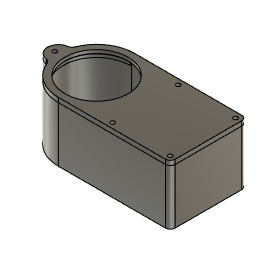
ad_extbox_alarm v14 (Autodesk Fusion 360 design; units mm, degrees)
Autodesk Fusion 360 part; units mm, degrees
note: some values were not read from the file. Set by a fixed rule: which face or edge a step refers to.
sketch "Sketch1" plane through (0, 0, 0) normal (0, 0, 1) x (1, 0, 0)
  circle A0 centre (0, 0) radius 31.5
  line L0 (-0.0628, 31.4999) -> (92.4372, 31.4999)
  line L1 (92.4372, 31.4999) -> (92.4372, -31.5001)
  line L2 (92.4372, -31.5001) -> (-0.0628, -31.5001)
  line L3 (-0.0628, -31.5001) -> (-0.0628, 31.4999)
  circle A1 centre (71.4372, -0.0001) radius 11
  circle A2 centre (26.4372, 24.9999) radius 1.75
  circle A3 centre (26.4372, -25.0001) radius 1.75
  circle A4 centre (71.4372, -25.0001) radius 1.75
  circle A5 centre (71.4372, 24.9999) radius 1.75
  circle A6 centre (0, 0) radius 26.15
  circle A7 centre (92.4372, 31.4999) radius 10.8
  circle A8 centre (92.4372, -31.5001) radius 10.8
  circle A9 centre (40.4372, -31.5001) radius 9
  circle A10 centre (40.4372, 31.4999) radius 9
  line L4 (40.4372, 26.9999) -> (87.9372, 26.9999)
  line L5 (87.9372, 26.9999) -> (87.9372, -27.0001)
  line L6 (87.9372, -27.0001) -> (40.4372, -27.0001)
  line L7 (40.4372, -27.0001) -> (40.4372, 26.9999)
  circle A11 centre (40.4372, -27.0001) radius 1.75
  circle A12 centre (87.9372, -27.0001) radius 1.75
  circle A13 centre (87.9372, 26.9999) radius 1.75
  circle A14 centre (40.4372, 26.9999) radius 1.75
  line L8 (57.4372, -24.8001) -> (77.4372, -24.8001)
  line L9 (77.4372, -24.8001) -> (77.4372, -28.8001)
  line L10 (77.4372, -28.8001) -> (57.4372, -28.8001)
  line L11 (57.4372, -28.8001) -> (57.4372, -24.8001)
  line L12 (57.4372, 28.7999) -> (77.4372, 28.7999)
  line L13 (77.4372, 28.7999) -> (77.4372, 24.7999)
  line L14 (77.4372, 24.7999) -> (57.4372, 24.7999)
  line L15 (57.4372, 24.7999) -> (57.4372, 28.7999)
  line L16 (85.7372, 9.9999) -> (89.7372, 9.9999)
  line L17 (89.7372, 9.9999) -> (89.7372, -10.0001)
  line L18 (89.7372, -10.0001) -> (85.7372, -10.0001)
  line L19 (85.7372, -10.0001) -> (85.7372, 9.9999)
  circle A15 centre (0, 0) radius 28.8
  circle A16 centre (0, 0) radius 27.75
  circle A17 centre (-31.5, 0.013) radius 9
  circle A18 centre (-34.5, 0.0043) radius 1.75
  circle A19 centre (-34.5, 0.0043) radius 2
  circle A20 centre (40.4372, 26.9999) radius 2
  circle A21 centre (87.9372, 26.9999) radius 2
  circle A22 centre (87.9372, -27.0001) radius 2
  circle A23 centre (40.4372, -27.0001) radius 2
  dimension "d1" = 63
  dimension "d6" = 92.5
  dimension "d7" = 63
  dimension "d8" = 22
  dimension "d9" = 21
  dimension "d11" = 31.5
  dimension "d12" = 3.5
  dimension "d13" = 3.5
  dimension "d14" = 3.5
  dimension "d15" = 3.5
  dimension "d16" = 21
  dimension "d18" = 21
  dimension "d19" = 50
  dimension "d21" = 6.5
  dimension "d22" = 6.5
  dimension "d23" = 50
  dimension "d24" = 45
  dimension "d26" = 45
  dimension "d36" = 52.3
  dimension "d44" = 21.6
  dimension "d45" = 21.6
  dimension "d46" = 18
  dimension "d47" = 18
  dimension "d48" = 52
  dimension "d50" = 52
  dimension "d53" = 4.5
  dimension "d54" = 4.5
  dimension "d55" = 4.5
  dimension "d56" = 52
  dimension "d57" = 3.5
  dimension "d58" = 3.5
  dimension "d59" = 3.5
  dimension "d60" = 3.5
  dimension "d78" = 20
  dimension "d79" = 4
  dimension "d80" = 2.7
  dimension "d81" = 15
  dimension "d82" = 20
  dimension "d83" = 4
  dimension "d84" = 2.7
  dimension "d85" = 15
  dimension "d86" = 4
  dimension "d87" = 20
  dimension "d88" = 2.7
  dimension "d89" = 21.5
  dimension "d95" = 57.6
  dimension "d96" = 55.5
  dimension "d100" = 18
  dimension "d101" = 3.5
  dimension "d102" = 3
  dimension "d106" = 4
  dimension "d107" = 4
  dimension "d108" = 4
  dimension "d109" = 4
  dimension "d110" = 4
  constraint coincident A0.centre A6.centre
  constraint horizontal L0
  constraint vertical L1
  constraint horizontal L2
  constraint vertical L3
  constraint coincident A0 L0.start
  constraint coincident L0.end L1.start
  constraint coincident L1.end L2.start
  constraint coincident L2 A9.centre
  constraint coincident L0 A10.centre
  constraint horizontal L4
  constraint vertical L5
  constraint horizontal L6
  constraint vertical L7
  constraint coincident L6.end L7.start
  constraint coincident L5.end L6.start
  constraint coincident L4.end L5.start
  constraint coincident L4.start L7.end
  constraint horizontal L8
  constraint vertical L9
  constraint horizontal L10
  constraint vertical L11
  constraint horizontal L12
  constraint vertical L13
  constraint horizontal L14
  constraint vertical L15
  constraint horizontal L16
  constraint vertical L17
  constraint horizontal L18
  constraint vertical L19
  constraint concentric A6 A15
  constraint concentric A6 A16
  constraint coincident A0 A17.centre
  constraint concentric A18 A19
  constraint concentric A13 A21
  constraint concentric A12 A22
  measures "d1" diameter of A0
  measures "d6" distance of L0.start L0.end
  measures "d7" distance of L0.start L2.end
  measures "d8" diameter of A1
  measures "d9" distance of L1 A1.centre
  measures "d11" distance of L2 A1.centre
  measures "d12" diameter of A2
  measures "d13" diameter of A3
  measures "d14" diameter of A4
  measures "d15" diameter of A5
  measures "d16" distance of L1 A5.centre
  measures "d18" distance of L1 A4.centre
  measures "d19" distance of A4.centre A5.centre
  measures "d21" distance of L2 A4.centre
  measures "d22" distance of L2 A3.centre
  measures "d23" vertical distance of A2.centre A3.centre
  measures "d24" distance of A2.centre A5.centre
  measures "d26" distance of A3.centre A4.centre
  measures "d36" diameter of A6
  measures "d44" diameter of A7
  measures "d45" diameter of A8
  measures "d46" diameter of A9
  measures "d47" diameter of A10
  measures "d48" distance of L1.end A9.centre
  measures "d50" distance of L0.end A10.centre
  measures "d53" distance of L1 L5
  measures "d54" distance of L2 L6
  measures "d55" distance of L0 L4
  measures "d56" distance of L1 L7
  measures "d57" diameter of A11
  measures "d58" diameter of A12
  measures "d59" diameter of A13
  measures "d60" diameter of A14
  measures "d78" distance of L8.start L8.end
  measures "d79" distance of L8.start L10.end
  measures "d80" distance of L2 L10
  measures "d81" distance of L1 L9
  measures "d82" distance of L12.start L12.end
  measures "d83" distance of L12.start L14.end
  measures "d84" distance of L0 L12
  measures "d85" distance of L1 L13
  measures "d86" distance of L16.start L16.end
  measures "d87" distance of L16.start L18.end
  measures "d88" distance of L1 L17
  measures "d89" distance of L2 L18
  measures "d95" diameter of A15
  measures "d96" diameter of A16
  measures "d100" diameter of A17
  measures "d101" diameter of A18
  measures "d102" distance of A17.centre A18.centre
  measures "d106" diameter of A19
  measures "d107" diameter of A20
  measures "d108" diameter of A21
  measures "d109" diameter of A22
  measures "d110" diameter of A23
extrude "Extrude1" add sketch "Sketch1" along normal blind 45.5 contours A0 L3 A15 | A0 L3 A15 A17 | A0 L0 L2 A9 A10 L7 | A0 L3 A15 A17 | A0 A15 A17 | L0 A10 L4 L7 A20 | L3 A15 A16 | L3 A15 A16 A17 | L2 A9 L6 L7 A23 | L3 A15 A16 A17 | A15 A16 A17 | L0 A7 A10 L4 L12 L13 L15 | A10 L4 L7 A20 | A4 A5 A7 A8 A9 A10 L4 L5 L6 L7 L8 L9 L11 L13 L14 L15 L16 L18 L19 | L3 A6 A16 | L3 A6 A16 A17 | L2 A8 A9 L6 L9 L10 L11 | A9 L6 L7 A23 | L3 A6 A16 A17 | A6 A16 A17 | L0 L1 A7 L4 L5 A21 | L4 L7 A14 A20 | L4 L7 A14 A20 | L3 A6 | L3 A6 A17 | L1 L2 A8 L5 L6 A22 | L6 L7 A11 A23 | L6 L7 A11 A23 | A6 A17 | A7 L4 L5 A21 | L4 L12 L13 L15 | A5 L4 L13 L14 L15 | L4 L7 A14 | L4 L7 A14 | A8 L5 L6 A22 | A4 L6 L8 L9 L11 | L6 L9 L10 L11 | L6 L7 A11 | L6 L7 A11 | L1 A7 A8 L5 L16 L17 L18 | L4 L5 A13 A21 | L4 L5 A13 A21 | L5 L6 A12 A22 | L5 L6 A12 A22 | L5 L16 L17 L18 | L5 L16 L18 L19 | L4 L5 A13 | L4 L5 A13 | A5 L14 | A5 L14 | L5 L6 A12 | L5 L6 A12 | A4 L8 | A4 L8 | A1 | A2 | A3 makes body 1
shell "Shell1" thickness 2.5 removed faces 1 at (63.7705, -6.9001, 45.5) on bodies 1
extrude "Extrude2" cut sketch "Sketch1" along normal blind 3.5 contours A5 L14 | A5 L14 | A4 L8 | A4 L8 | A1 | A2 | A3 bodies 1
sketch "Sketch2" plane through (0, -31.5001, 0) normal (0, -1, 0) x (1, 0, 0)
  line L0 (92.4372, 45.5) -> (-0.0628, 45.5)
  line L1 (-0.0628, 45.5) -> (-0.0628, 0)
  line L2 (-0.0628, 0) -> (92.4372, 0)
  line L3 (31.4372, 45.5) -> (121.4372, 45.5)
  line L4 (121.4372, 45.5) -> (121.4372, 27.5)
  line L5 (121.4372, 27.5) -> (31.4372, 27.5)
  line L6 (31.4372, 27.5) -> (31.4372, 45.5)
  line L7 (92.4372, 0) -> (92.4372, 45.5)
  dimension "d37" = 90
  dimension "d38" = 18
  dimension "d39" = 31.5
  constraint horizontal L3
  constraint vertical L4
  constraint horizontal L5
  constraint vertical L6
  constraint coincident L0 L3.start
  measures "d37" distance of L3.start L3.end
  measures "d38" distance of L3.start L5.end
  measures "d39" distance of L1 L6
extrude "Extrude4" add sketch "Sketch1" along normal blind 45.5 contours A0 A17 | L0 A10 L4 L7 A20 | L2 A9 L6 L7 A23 | A10 L4 L7 A20 | A9 L6 L7 A23 | L0 L1 A7 L4 L5 A21 | L4 L7 A14 A20 | L4 L7 A14 A20 | L1 L2 A8 L5 L6 A22 | L6 L7 A11 A23 | L6 L7 A11 A23 | A7 L4 L5 A21 | L4 L7 A14 | L4 L7 A14 | A8 L5 L6 A22 | L6 L7 A11 | L6 L7 A11 | L4 L5 A13 A21 | L4 L5 A13 A21 | L5 L6 A12 A22 | L5 L6 A12 A22 | L4 L5 A13 | L4 L5 A13 | L5 L6 A12 | L5 L6 A12 | A18 | A19 bodies 1
extrude "Extrude5" cut sketch "Sketch1" against normal blind 20 from surface at 45.5 contours L4 L7 A14 A20 | L4 L7 A14 A20 | L6 L7 A11 A23 | L6 L7 A11 A23 | L4 L7 A14 | L4 L7 A14 | L6 L7 A11 | L6 L7 A11 | L4 L5 A13 A21 | L4 L5 A13 A21 | L5 L6 A12 A22 | L5 L6 A12 A22 | L4 L5 A13 | L4 L5 A13 | L5 L6 A12 | L5 L6 A12 | A18 | A19 bodies 1
extrude "Extrude6" add sketch "Sketch1" along normal blind 3.75 from surface at 45.5 separate body contours A0 L3 A15 | A0 L3 A15 A17 | A0 L0 L2 A9 A10 L7 | A0 L3 A15 A17 | A0 A15 A17 | A0 A17 | L0 A10 L4 L7 A20 | L3 A15 A16 | L3 A15 A16 A17 | L2 A9 L6 L7 A23 | L3 A15 A16 A17 | A15 A16 A17 | L0 A7 A10 L4 L12 L13 L15 | A10 L4 L7 A20 | A4 A5 A7 A8 A9 A10 L4 L5 L6 L7 L8 L9 L11 L13 L14 L15 L16 L18 L19 | L3 A6 A16 | L3 A6 A16 A17 | L2 A8 A9 L6 L9 L10 L11 | A9 L6 L7 A23 | L3 A6 A16 A17 | A6 A16 A17 | L0 L1 A7 L4 L5 A21 | L4 L7 A14 A20 | L4 L7 A14 A20 | L3 A6 | L3 A6 A17 | L1 L2 A8 L5 L6 A22 | L6 L7 A11 A23 | L6 L7 A11 A23 | A6 A17 | A7 L4 L5 A21 | L4 L12 L13 L15 | A5 L4 L13 L14 L15 | A8 L5 L6 A22 | A4 L6 L8 L9 L11 | L6 L9 L10 L11 | L1 A7 A8 L5 L16 L17 L18 | L4 L5 A13 A21 | L4 L5 A13 A21 | L5 L6 A12 A22 | L5 L6 A12 A22 | L5 L16 L17 L18 | L5 L16 L18 L19 | A5 L14 | A5 L14 | A4 L8 | A4 L8 | A1 | A2 | A3 | A19 makes body 2
fillet "Fillet1" radius 4 2 edges at (92.4372, -31.5001, 22.75) (92.4372, 31.4999, 22.75) on bodies 1 2
fillet "Fillet1" radius 4 2 edges at (92.4372, -31.5001, 47.375) (92.4372, 31.4999, 47.375) on bodies 1 2
extrude "Extrude7" cut sketch "Sketch1" along normal blind 20 from surface at 45.5 contours L3 A6 | L3 A6 A17 | A6 A17 bodies 2
fillet "Fillet2" radius 1 1 edges at (-24.3804, -9.4562, 45.5) on bodies 2
extrude "Extrude8" add sketch "Sketch1" against normal blind 3 from surface at 45.5 contours L4 L12 L13 L15 | A5 L4 L13 L14 L15 | A4 L6 L8 L9 L11 | L6 L9 L10 L11 | L5 L16 L17 L18 | L5 L16 L18 L19 | A5 L14 | A4 L8 picked at (71.8759, 25.4541) picked at (71.3204, -25.46) bodies 2
fillet "Fillet3" radius 0.7 12 edges at (67.4372, -28.8001, 42.5) (57.4372, -26.8001, 42.5) (67.4372, -24.8001, 42.5) (77.4372, -26.8001, 42.5) (85.7372, -0.0001, 42.5) (87.7372, -10.0001, 42.5) (89.7372, -0.0001, 42.5) (87.7372, 9.9999, 42.5) (67.4372, 24.7999, 42.5) (77.4372, 26.7999, 42.5) (67.4372, 28.7999, 42.5) (57.4372, 26.7999, 42.5) on bodies 2
extrude "Extrude9" add sketch "Sketch1" against normal blind 3 from surface at 45.5 contours L3 A15 A16 A17 | L3 A15 A16 A17 | A15 A16 A17 bodies 2
fillet "Fillet4" radius 4 4 edges at (-30.218, -8.8952, 22.75) (-30.2106, 8.9202, 22.75) (-30.218, -8.8952, 47.375) (-30.2106, 8.9202, 47.375) on bodies 1 2
equation "d1 = alarm_d + wall * 2"
equation "alarm_d = 58 mm"
equation "wall = 2.5 mm"
equation "connector_d = 22 mm"
equation "box_w = 90 mm"
equation "d6 = box_w + wall"
equation "d7 = alarm_d + wall * 2"
equation "d8 = connector_d"
equation "d9 = c_offset"
equation "mount_d = 3.5 mm"
equation "d11 = alarm_d / 2 + wall"
equation "d12 = mount_d"
equation "d13 = mount_d"
equation "d14 = mount_d"
equation "d15 = mount_d"
equation "d16 = c_offset"
equation "c_offset = connector_d / 2 + 10 mm"
equation "d18 = c_offset"
equation "d19 = mount_y"
equation "mount_y = 50 mm"
equation "d21 = ( alarm_d + wall * 2 - mount_y ) / 2"
equation "d22 = ( alarm_d + wall * 2 - mount_y ) / 2"
equation "d23 = mount_y"
equation "d24 = mount_x"
equation "mount_x = 45 mm"
equation "d26 = mount_x"
equation "box_h = 43 mm"
equation "d28 = box_h + wall"
equation "d32 = wall"
equation "d33 = wall + 1 mm"
equation "alarm_r_d = 52.3 mm"
equation "d36 = alarm_r_d"
equation "d37 = box_w"
equation "d38 = box_h - box_l_h"
equation "d39 = alarm_d / 2 + wall"
equation "box_l_h = 25 mm"
equation "cmount_d = 18 mm"
equation "d44 = cmount_d * 1.2"
equation "d45 = cmount_d * 1.2"
equation "d46 = cmount_d"
equation "d47 = cmount_d"
equation "d48 = cmount_x"
equation "cmount_x = 52 mm"
equation "d50 = cmount_x"
equation "d51 = box_h + wall"
equation "d53 = cmount_off"
equation "d54 = cmount_off"
equation "d55 = cmount_off"
equation "d56 = cmount_x"
equation "d57 = mount_d"
equation "d58 = mount_d"
equation "d59 = mount_d"
equation "d60 = mount_d"
equation "cmount_off = mount_d + 1 mm"
equation "d66 = wall * 1.5"
equation "border_w = 4 mm"
equation "border_l = 20 mm"
equation "border_offset = wall + 0.2 mm"
equation "d78 = border_l"
equation "d79 = border_w"
equation "d80 = border_offset"
equation "d82 = border_l"
equation "d83 = border_w"
equation "d84 = border_offset"
equation "d86 = border_w"
equation "d87 = border_l"
equation "d88 = border_offset"
equation "d89 = ( alarm_d + wall * 2 - border_l ) / 2"
equation "d95 = alarm_d + wall * 2 - border_offset * 2"
equation "d96 = alarm_r_d + 3.2 mm"
equation "d100 = cmount_d"
equation "d101 = mount_d"
equation "mount_h_d = 4 mm"
equation "d106 = mount_h_d"
equation "d107 = mount_h_d"
equation "d108 = mount_h_d"
equation "d109 = mount_h_d"
equation "d110 = mount_h_d"
named bodies: "ade_alarm_case", "ade_alarm_top"
